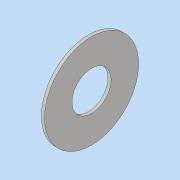
# Autodesk Inventor part: WasherForThread_5_16_18
Saved by Autodesk Inventor 2017 (Build 210142000, 142)
## iProperties
Created: 2016-11-27
Part Number: WasherForThread_5_16_18
Material: Generic
Document SubType Name: Modeling
Designer: techn
Density: 1 g/cm^3
Appearance: Default
Author: techn
Autodesk Inventor part; units mm, degrees
ref_plane "YZ Plane" through (0, 0, 0) normal (1, 0, 0) x (0, 1, 0)
ref_plane "XZ Plane" through (0, 0, 0) normal (0, 1, 0) x (-1, 0, 0)
ref_plane "XY Plane" through (0, 0, 0) normal (0, 0, 1) x (1, 0, 0)
sketch "Sketch1" plane through (0, 0, 0) normal (0, 0, 1) x (1, 0, 0)
  line L0 (0, 0) -> (0, 3.9624)
  line L1 (0, 0) -> (0, 9.525)
  line L2 (0, 9.525) -> (0.635, 9.525)
  line L3 (0.635, 9.525) -> (0.635, 3.9624)
  line L4 (0.635, 3.9624) -> (0, 3.9624)
  line L5 (0, 0) -> (4.048, 0)
  line L6 (0, 9.525) -> (0.635, 9.525)
  line L7 (0.635, 9.525) -> (0.635, 3.9624)
  line L8 (0.635, 3.9624) -> (0, 3.9624)
  line L9 (0, 3.9624) -> (0, 9.525)
  dimension "d3" = 3.9624
  dimension "d4" = 9.525
  dimension "d5" = 0.635
  constraints: 20 end point, 4 perpendicular, 2 horizontal, 2 parallel, 2 vertical
  measures "d3" distance of L0.start L0.end
  measures "d4" distance of L0.start L1.end
  measures "d5" distance of L1.end L2.end
revolve "Revolution1" add sketch "Sketch1" angle 360 about axis through (0, 0, 0) along (1, 0, 0)
body "Solid1"
